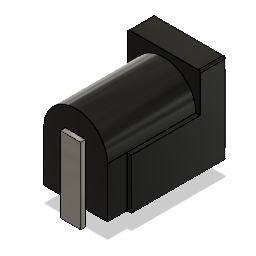
DCJack (Autodesk Fusion 360 design; units mm, degrees)
Autodesk Fusion 360 part; units mm, degrees
note: some values were not read from the file. Chosen so that the rebuilt part matches the saved one: a direction; which face or edge a step refers to.
sketch "Sketch1" plane through (0, 0, 0) normal (0, 1, 0) x (1, 0, 0) in component "DC Jack"
  line L0 (0, 0) -> (9, 0)
  line L1 (9, 0) -> (9, -11)
  line L2 (9, -11) -> (0, -11)
  line L3 (0, -11) -> (0, 0)
  dimension "d1" = 9
  dimension "d2" = 11
  measures "d1" distance of L0.start
  measures "d2" distance of L0.start
extrude "Extrude1" add sketch "Sketch1" along normal blind 3.3 makes body 1 in component "DC Jack"
sketch "Sketch2" plane through (0, 3.3, 0) normal (0, 1, 0) x (-1, 0, 0) in component "DC Jack"
  line L0 (0, 11) -> (-9, 11)
  line L1 (-9, 11) -> (-9, 0)
  line L2 (-9, 0) -> (0, 0)
  line L3 (0, 0) -> (0, 11)
  circle A0 centre (-4.5, 4.75) radius 3.95
  line L4 (-4.5, 0) -> (-4.5, 0.8) construction
  line L5 (-9, 4.75) -> (-8.45, 4.75)
  line L6 (0, 4.75) -> (-0.55, 4.75)
  dimension "d5" = 0.8
  dimension "d6" = 7.9
  measures "d6" diameter of A0
extrude "Extrude2" add sketch "Sketch2" along normal blind 8.5 contours L0 L1 L3 A0 L5 L6 | A0 bodies 1 in component "DC Jack"
sketch "Sketch3" plane through (0, 11.8, 0) normal (0, 1, 0) x (-1, 0, 0) in component "DC Jack"
  line L0 (0, 11) -> (-9, 11)
  line L1 (-9, 11) -> (-9, 4.75)
  line L2 (-9, 4.75) -> (-8.45, 4.75)
  arc A0 (-8.45, 4.75) -> (-0.55, 4.75) centre (-4.5, 4.75) ccw
  line L3 (-0.55, 4.75) -> (0, 4.75)
  line L4 (0, 4.75) -> (0, 11)
  line L5 (-0.55, 4.75) -> (-0.55, 11)
  line L6 (-8.45, 4.75) -> (-8.45, 11)
extrude "Extrude3" add sketch "Sketch3" along normal blind 2.4 contours L0 A0 L5 L6 bodies 1 in component "DC Jack"
sketch "Sketch4" plane through (0, 0, 0) normal (0, -1, 0) x (1, 0, 0) in component "DC Jack"
  line L0 (9, 11) -> (0, 11)
  line L1 (0, 11) -> (0, 0)
  line L2 (0, 0) -> (9, 0)
  line L3 (9, 0) -> (9, 11)
hole "Hole1" at (4.5, 0, 4.75) direction (0, 1, 0) diameter 6.5 depth 9.6 tip angle 180 bodies 1 in component "DC Jack"
sketch "Sketch1 (2)" plane through (0, 9.6, 0) normal (0, -1, 0) x (1, 0, 0) in component "Connection"
  circle A0 centre (4.5, 4.75) radius 3.25
  circle A1 centre (4.5, 4.75) radius 1.25
  dimension "d14" = 2.5
  measures "d14" diameter of A1
extrude "Extrude1'" add sketch "Sketch1 (2)" along normal blind 8.1 separate body contours A1 makes body 2 in component "Connection"
ref_plane "WorkPlane1" through (1.2501, 0.7141, 4.7724) normal (0.999976, 0, -0.006903) x (0.006903, 0, 0.999976) in component "Connection"
ref_plane "WorkPlane2" through (3.2501, 2.383, 4.7654) normal (-0.999924, 0, 0.012358) x (0.012358, 0, 0.999924) in component "Connection"
ref_plane "WorkPlane3" through (2.2501, 2.383, 4.7764) normal (-0.999954, 0, 0.009631) x (0.009631, 0, 0.999954) in component "Connection"
sketch "Sketch2 (2)" plane through (2.2501, 2.383, 4.7764) normal (-0.999954, 0, 0.009631) x (0.009631, 0, 0.999954) in component "Connection"
  line L0 (0.0386, 0.917) -> (-4.7112, 0.917)
  line L1 (-2.5152, 0.917) -> (-2.5152, 2.9)
  line L2 (-2.5152, 2.9) -> (-1.4, 4.1)
  line L3 (-1.4, 4.1) -> (-2.5152, 5.8045)
  line L4 (-2.5152, 5.8045) -> (-2.6321, 5.728)
  line L5 (-2.6321, 5.728) -> (-1.567, 4.1)
  line L6 (-1.567, 4.1) -> (-2.6321, 2.9477)
  line L7 (-2.6321, 2.9477) -> (-2.6321, 0.917)
extrude "Extrude2'" add sketch "Sketch2 (2)" against normal blind 4.54 separate body makes body 3 in component "Connection"
move_body "Move1" bodies 3 to x (1, 0, 0) y (0, -1, 0) z (0, 0, -1) at (0.0109, 10.8142, 9.4015) in component "Connection"
fillet "Fillet1" radius 0.25 5 edges at (0, 0, 5.5) (0, 1.65, 0) (4.5, 0, 0) (9, 1.65, 0) (9, 0, 5.5) on bodies 1 in component "DC Jack"
chamfer "Chamfer1" distance 0.25 angle 45 1 edges at (5.6753, 0, 7.7801) on bodies 1 in component "DC Jack"
fillet "Fillet1'" radius 1 1 edges at (3.3346, 1.5, 4.298) on bodies 2 in component "Connection"
sketch "Sketch3 (2)" plane through (0, 0, 0) normal (-1, 0, 0) x (0, 0, 1) in component "Connection"
  line L0 (0.25, 3.3) -> (0.25, 0.25)
  line L1 (0.25, 0.25) -> (11, 0.25)
  line L2 (11, 0.25) -> (11, 11.8)
  line L3 (11, 11.8) -> (4.75, 11.8)
  line L4 (4.75, 11.8) -> (4.75, 3.3)
  line L5 (4.75, 3.3) -> (0.25, 3.3)
  line L6 (4.75, 11.8) -> (12.85, 11.8)
  line L7 (12.85, 11.8) -> (12.85, 9.7)
  line L8 (12.85, 9.7) -> (4.75, 9.7)
  line L9 (4.75, 9.7) -> (4.75, 11.8)
  dimension "d24" = 2.1
  dimension "d25" = 8.1
extrude "Extrude3'" add sketch "Sketch3 (2)" along normal blind 0.6 separate body contours L2 L3 L4 L6 L8 L9 | L2 L6 L7 L8 makes body 4 in component "Connection"
sketch "Sketch4 (2)" plane through (0, 14.2, 0) normal (0, 1, 0) x (-1, 0, 0) in component "Connection"
  line L0 (-0.55, 4.75) -> (-0.55, 11)
  line L1 (-0.55, 11) -> (-8.45, 11)
  line L2 (-8.45, 11) -> (-8.45, 4.75)
  arc A0 (-8.45, 4.75) -> (-0.55, 4.75) centre (-4.5, 4.75) ccw
  line L3 (-3.25, 3.5) -> (-5.75, 3.5)
  line L4 (-5.75, 3.5) -> (-5.75, 12.8738)
  line L5 (-5.75, 12.8738) -> (-3.25, 12.8738)
  line L6 (-3.25, 12.8738) -> (-3.25, 3.5)
  circle A1 centre (-4.5, 4.75) radius 1.25
extrude "Extrude4" add sketch "Sketch4 (2)" along normal blind 0.6 separate body contours L1 L4 L6 A1 | L1 L4 L5 L6 | A1 | L3 L6 A1 | L3 L4 A1 makes body 5 in component "Connection"
sketch "Sketch5" plane through (0, 0, 11) normal (0, 0, 1) x (1, 0, 0) in component "Connection"
  arc A0 (8.75, 0) -> (9, 0.25) centre (8.75, 0.25) ccw
  line L0 (9, 0.25) -> (9, 11.8)
  line L1 (9, 11.8) -> (8.45, 11.8)
  line L2 (8.45, 11.8) -> (8.45, 14.2)
  line L3 (8.45, 14.2) -> (0.55, 14.2)
  line L4 (0.55, 14.2) -> (0.55, 11.8)
  line L5 (0.55, 11.8) -> (0, 11.8)
  line L6 (0, 11.8) -> (0, 0.25)
  arc A1 (0, 0.25) -> (0.25, 0) centre (0.25, 0.25) ccw
  line L7 (0.25, 0) -> (8.75, 0)
  line L8 (4.5, 14.2) -> (4.5, 9.8) construction
  line L9 (3.45, 9.8) -> (5.55, 9.8)
  line L10 (5.55, 9.8) -> (5.55, 9.2)
  line L11 (5.55, 9.2) -> (3.45, 9.2)
  line L12 (3.45, 9.2) -> (3.45, 9.8)
  dimension "d30" = 4.4
  dimension "d31" = 2.1
  dimension "d32" = 0.6
extrude "Extrude5" add sketch "Sketch5" along normal up to surface (1.8738 mm away) separate body contours L9 L10 L11 L12 makes body 6 in component "Connection"
component "DC Jack" placed x (1, 0, 0) y (0, 0, 1) z (0, -1, 0) at (0, 10.9268, -0.8359)
component "Connection" placed x (1, 0, 0) y (0, 1, 0) z (0, 0, 1) at (0, 0, 0) in component "DC Jack"
equation "d15 = 9.60 mm - 1.5 mm"
equation "d19 = -2.27 mm * 2"
